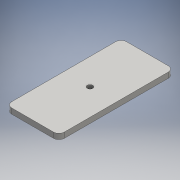
# Autodesk Inventor part: Phone Mount
Saved by Autodesk Inventor 2016 (Build 200138000, 138)
## iProperties
Created: 2015-09-05
Part Number: Phone Mount
Material: Generic
Document SubType Name: Modeling
Designer: Tim
Density: 1 g/cm^3
Appearance: Default
Author: Tim
Autodesk Inventor part; units mm, degrees
ref_plane "YZ Plane" through (0, 0, 0) normal (1, 0, 0) x (0, 1, 0)
ref_plane "XZ Plane" through (0, 0, 0) normal (0, 1, 0) x (-1, 0, 0)
ref_plane "XY Plane" through (0, 0, 0) normal (0, 0, 1) x (1, 0, 0)
sketch "Sketch1" plane through (0, 0, 0) normal (0, 0, 1) x (1, 0, 0)
  line L0 (46.04, 0) -> (0, 0)
  arc A0 (-6, 6) -> (0, 0) centre (0, 6) ccw
  line L1 (-6, 6) -> (-6, 120.62)
  arc A1 (46.04, 0) -> (52.04, 6) centre (46.04, 6) ccw
  line L2 (52.04, 120.62) -> (52.04, 6)
  arc A2 (0, 126.62) -> (-6, 120.62) centre (0, 120.62) ccw
  line L3 (0, 126.62) -> (46.04, 126.62)
  arc A3 (52.04, 120.62) -> (46.04, 126.62) centre (46.04, 120.62) ccw
  constraints: 8 end point, 8 point on circle, 4 centre point
extrude "Extrusion1" add sketch "Sketch1" along normal mid plane 6
sketch "Sketch2" plane through (0, 0, 3) normal (0, 0, 1) x (1, 0, 0)
  line L0 (0, 0) -> (46.04, 0) projected
  line L1 (0, 126.62) -> (46.04, 126.62) projected
  point P0 (23.02, 63.31)
hole "Hole1" at (23.02, 63.31, 3) direction (0, 0, -1) diameter 3.7 end through all counterbore diameter 6 counterbore depth 3.5
body "Solid1"
